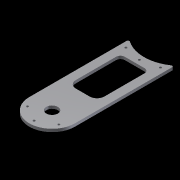
# Autodesk Inventor part: JointC2cover_2nd
Saved by Autodesk Inventor 2011 SP1 (Build 150282100, 282)
## iProperties
Created: 2013-02-08
Part Number: JointC2cover_2nd
Document SubType Name: Modeling
Designer: arihon
Density: 1 g/cm^3
Author: arihon
Autodesk Inventor part; units mm, degrees
ref_plane "YZ Plane" through (0, 0, 0) normal (1, 0, 0) x (0, 1, 0)
ref_plane "XZ Plane" through (0, 0, 0) normal (0, 1, 0) x (-1, 0, 0)
ref_plane "XY Plane" through (0, 0, 0) normal (0, 0, 1) x (1, 0, 0)
sketch "スケッチ1" plane through (0, 0, 0) normal (0, 0, 1) x (1, 0, 0)
  circle A0 centre (-10.8253, -50.5) radius 0.7835
  circle A1 centre (0, -56.75) radius 0.7835
  circle A2 centre (10.8253, -50.5) radius 0.7835
  circle A3 centre (11.9284, 18.6695) radius 0.7835
  circle A4 centre (0, 16.025) radius 0.7835
  circle A5 centre (-11.9284, 18.6695) radius 0.7835
  line L0 (-9.85, -18.05) -> (-9.85, 9.75)
  arc A6 (-6.8, 12.8) -> (-9.85, 9.75) centre (-6.8, 9.75) ccw
  line L1 (-6.8, 12.8) -> (6.8, 12.8)
  arc A7 (9.85, 9.75) -> (6.8, 12.8) centre (6.8, 9.75) ccw
  line L2 (9.85, 9.75) -> (9.85, -18.05)
  arc A8 (4.8, -23.1) -> (9.85, -18.05) centre (4.8, -18.05) ccw
  line L3 (4.8, -23.1) -> (-4.8, -23.1)
  arc A9 (-9.85, -18.05) -> (-4.8, -23.1) centre (-4.8, -18.05) ccw
  circle A10 centre (0, -44.25) radius 4
  arc A11 (-15.75, 24.8351) -> (15.75, 24.8351) centre (0, 44.25) ccw
  line L4 (-15.75, -44.25) -> (-15.75, 24.8351)
  arc A12 (-15.75, -44.25) -> (15.75, -44.25) centre (0, -44.25) ccw
  line L5 (15.75, 24.8351) -> (15.75, -44.25)
  point P0 (0, 0)
  point P1 (0, 0)
  constraints: 13 centre point, 12 end point, 12 point on circle
extrude "押し出し1" add sketch "スケッチ1" along normal blind 2
fillet "フィレット1" radius 1 2 edges at (-15.75, 24.8351, 1) (15.75, 24.8351, 1)
